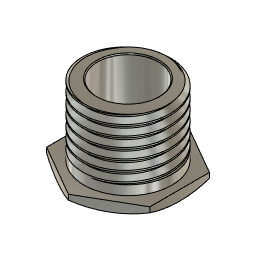
A-1122 nut (Autodesk Fusion 360 design; units mm, degrees)
Autodesk Fusion 360 part; units mm, degrees
sketch "Sketch1" plane through (0, 0, 0) normal (0, 0, 1) x (1, 0, 0)
  circle A0 centre (0, 0) radius 3.25
  line L0 (5.5, 3.1754) -> (0, 6.3509)
  line L1 (0, 6.3509) -> (-5.5, 3.1754)
  line L2 (-5.5, 3.1754) -> (-5.5, -3.1754)
  line L3 (-5.5, -3.1754) -> (0, -6.3509)
  line L4 (0, -6.3509) -> (5.5, -3.1754)
  line L5 (5.5, -3.1754) -> (5.5, 3.1754)
  dimension "d1" = 6.5
  dimension "d2" = 5.5
  constraint coincident A0.centre origin
  measures "d1" diameter of A0
  measures "d2" distance of A0.centre L5
extrude "Extrude1" add sketch "Sketch1" along normal blind 2
sketch "Sketch2" plane through (0, 0, 2) normal (0, 0, 1) x (-1, 0, 0)
  circle A0 centre (0, 0) radius 3.25
  circle A1 centre (0, 0) radius 4.65
  circle A2 centre (0, 0) radius 6.5
  dimension "d5" = 9.3
  constraint concentric A0 A1
  constraint concentric A1 A2
  measures "d5" diameter of A1
chamfer "Chamfer3" distance 0.2 angle 45 1 edges at (-3.0301, 1.1753, 0)
sketch "Sketch3" plane through (0, 0, 0) normal (1, 0, 0) x (0, 1, 0)
  line L0 (6.3509, 0) -> (6.3509, 2) construction
  line L1 (-6.3509, 0) -> (-6.3509, 2) construction
  line L2 (-10, 1.45) -> (9, 1.45) construction
  line L3 (0, -4.0186) -> (0, 32.4075)
  circle A0 centre (0, 14.1944) radius 18.213
  line L4 (3.25, 0.2) -> (-3.25, 0.2) construction
  line L5 (-3.25, 0.2) -> (-3.25, 0) construction
  line L6 (-3.25, 0) -> (3.25, 0) construction
  line L7 (3.25, 0) -> (3.25, 0.2) construction
  circle A1 centre (0, 10.9908) radius 11.4613
  dimension "d12" = 0.55
  constraint perpendicular L0 L2
  constraint perpendicular L2 L3
  constraint coincident A0 L3.end
  constraint coincident A0 L3.start
  constraint coincident L4.end L5.start
  constraint perpendicular L4 L5
  constraint perpendicular L5 L6
  constraint coincident L4.start L7.end
  constraint perpendicular L4 L7
  constraint coincident L5.end A1
  measures "d12" distance of L1.end L2
revolve "Revolve2" cut sketch "Sketch3" angle 360 about axis through (0, 0, -4.0186) along (0, 0, 1) contours L3 A0 A1 picked at (3.1181, 28.7424)
extrude "Extrude4" add sketch "Sketch2" along normal blind 7.497 contours A1
thread "Thread3" "ANSI Unified Screw Threads 0.375 3/8-24 UNF 1A" major diameter 9.3599 minor diameter 8.2372 pitch 1.0583 angle 60 modelled right hand crest width 0.1699 on face at (-4.6269, 0.463, 6.998) from (0, 0, 3) to (0, 0, 9.497) crest through (-4.6799, 0, 1.7354)
chamfer "Chamfer4" distance 0.1 angle 45 1 edges at (3.0301, -1.1753, 9.497)
equation "d3 = 9.5 mm - 7.5 mm"
equation "d23 = 7.497 mm - 1 mm"
